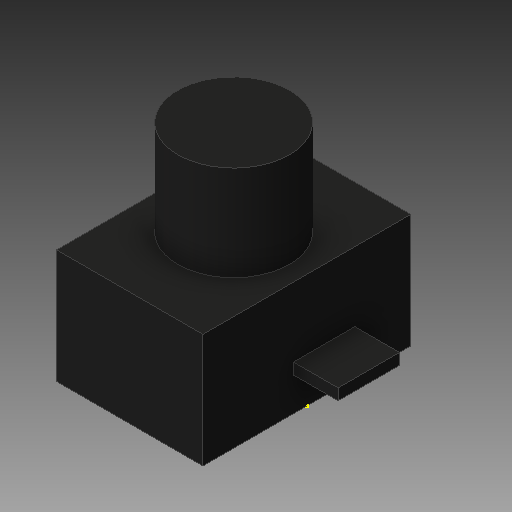
# Autodesk Inventor part: Camera
Saved by Autodesk Inventor 2018 (Build 220112000, 112)
## iProperties
Created: 2018-03-11
Part Number: Camera
Material: Generic
Document SubType Name: Modeling
Designer: Suchanek
Density: 1 g/cm^3
Appearance: Default
Mass: 3.17492 g
Surface Area: 14.5304 cm^2
Volume: 3.17492 cm^3
Author: Suchanek
Autodesk Inventor part; units mm, degrees
ref_plane "YZ Plane" through (0, 0, 0) normal (1, 0, 0) x (0, 1, 0)
ref_plane "XZ Plane" through (0, 0, 0) normal (0, 1, 0) x (-1, 0, 0)
ref_plane "XY Plane" through (0, 0, 0) normal (0, 0, 1) x (1, 0, 0)
sketch "Sketch1" plane through (0, 0, 0) normal (0, 1, 0) x (-1, 0, 0)
  line L0 (-6.55, 9.3) -> (6.55, 9.3)
  line L1 (6.55, 9.3) -> (6.55, -9.3)
  line L2 (6.55, -9.3) -> (-6.55, -9.3)
  line L3 (-6.55, -9.3) -> (-6.55, 9.3)
  line L4 (0, 0) -> (1, 0)
  line L5 (0, 0) -> (0, -1)
  dimension "d0" = 18.6
  dimension "d1" = 13.1
  dimension "d2" = 1
  dimension "d3" = 1
  constraints: 12 end point, 2 horizontal, 2 parallel, 1 perpendicular, 1 vertical, 2 other
  measures "d0" distance of L0.end L1.end
  measures "d1" distance of L1.end L2.end
  measures "d2" distance of L4.start L4.end
  measures "d3" distance of L4.start L5.end
extrude "Extrusion1" add sketch "Sketch1" along normal blind 10.2
sketch "Sketch2" plane through (0, 10.2, 0) normal (0, 1, 0) x (1, 0, 0)
  circle A0 centre (0, 0) radius 5
  dimension "d6" = 10
  constraints: 1 centre point, 1 coincident
  measures "d6" diameter of A0
extrude "Extrusion2" add sketch "Sketch2" along normal blind 8.5
sketch "Sketch3" plane through (6.55, 0, 9.3) normal (1, 0, 0) x (0, 0, -1)
  point P0 (9.3, 0)
sketch "Sketch4" plane through (6.55, 0, 9.3) normal (1, 0, 0) x (0, 0, -1)
  circle A0 centre (7.5, 3.5) radius 2.5
  line L0 (0, 0) -> (0, 10.2) projected
  line L1 (18.6, 0) -> (0, 0) projected
  point P0 (9.3, 0)
  dimension "d9" = 5
  dimension "d10" = 7.5
  dimension "d11" = 3.5
  constraints: 1 centre point
  measures "d9" diameter of A0
  measures "d10" distance from line of L0 A0.centre
  measures "d11" distance from line of L1 A0.centre
extrude "Extrusion3" [suppressed]
sketch "Sketch5" plane through (11.55, 3.5, 1.8) normal (1, 0, 0) x (0, 0, -1)
  circle A0 centre (0, 0) radius 15
  point P0 (1.8, -3.5)
  dimension "d14" = 30
  constraints: 1 centre point
  measures "d14" diameter of A0
extrude "Extrusion4" [suppressed]
sketch "Náčrt6" plane through (6.55, 0, 9.3) normal (1, 0, 0) x (0, 0, -1)
  line L0 (18.6, 0) -> (0, 0) projected
  line L1 (18.6, 0) -> (18.6, 10.2) projected
  line L2 (0, 10.2) -> (18.6, 10.2) projected
  line L3 (0, 0) -> (0, 10.2) projected
  line L4 (13.6, 3) -> (8.1, 3)
  line L5 (8.1, 3) -> (8.1, 4)
  line L6 (8.1, 4) -> (13.6, 4)
  line L7 (13.6, 4) -> (13.6, 3)
  point P0 (9.3, 0)
  dimension "d17" = 10.2
  dimension "d18" = 18.6
  dimension "d19" = 3
  dimension "d20" = 1
  dimension "d21" = 5.5
  dimension "d22" = 5
  constraints: 8 end point, 2 parallel, 1 horizontal, 1 perpendicular
  measures "d17" distance of L0.start L1.end
  measures "d18" distance of L0.start L0.end
  measures "d19" distance between parallel lines of L0 L4
  measures "d20" distance of L6.end L4.start
  measures "d21" distance of L4.start L4.end
  measures "d22" distance between parallel lines of L1 L7
extrude "Vysunutí5" add sketch "Náčrt6" along normal blind 4 contours L4 L5 L6 L7
body "Solid1"
